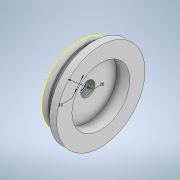
# Autodesk Inventor part: Крышка_пром_новая
Saved by Autodesk Inventor 2021 (Build 250183000, 183)
## iProperties
Created: 2023-04-26
Part Number: Крышка_пром_новая
Material: Типовые
Document SubType Name: Modeling
Designer: gdevc
Density: 1 g/cm^3
Appearance: По умолчанию
Mass: 23.6279 g
Surface Area: 96.7653 cm^2
Volume: 23.6279 cm^3
Author: gdevc
Autodesk Inventor part; units mm, degrees
ref_plane "YZ Plane" through (0, 0, 0) normal (1, 0, 0) x (0, 1, 0)
ref_plane "XZ Plane" through (0, 0, 0) normal (0, 1, 0) x (-1, 0, 0)
ref_plane "XY Plane" through (0, 0, 0) normal (0, 0, 1) x (1, 0, 0)
sketch "Эскиз1" plane through (0, 0, 0) normal (0, 0, 1) x (1, 0, 0)
  line L0 (0, 0) -> (0, 26)
  line L1 (10, 26.1456) -> (10, 30.5)
  line L2 (10, 30.5) -> (15, 30.5)
  line L3 (15, 30.5) -> (15, 20)
  line L4 (15, 20) -> (6, 20)
  line L5 (6, 20) -> (6, 0)
  line L6 (6, 0) -> (0, 0)
  line L7 (0, 26) -> (4.5, 26)
  line L8 (4.5, 26) -> (5, 25.5)
  line L9 (5, 25.5) -> (10, 25.5)
  line L10 (10, 25.5) -> (10, 26.1456)
  dimension "d1" = 52
  dimension "d2" = 0.5
  dimension "d3" = 45
  dimension "d4" = 5
  dimension "d5" = 15
  dimension "d6" = 6
  dimension "d7" = 40
  dimension "d8" = 4.5
  dimension "d23" = 10
  constraints: 22 end point, 6 perpendicular, 1 horizontal, 1 parallel, 1 vertical
  measures "d1" diameter of L7 L6
  measures "d2" distance between parallel lines of L7 L9
  measures "d3" angle of L7 L8
  measures "d4" distance of L8.end L9.end
  measures "d5" distance between parallel lines of L3 L0
  measures "d6" distance between parallel lines of L0 L5
  measures "d7" diameter of L4 L6
  measures "d8" distance between parallel lines of L7 L2
  measures "d23" distance between parallel lines of L0 L1
revolve "Вращение1" add sketch "Эскиз1" angle 360 about axis through (6, 0, 0) along (-1, 0, 0)
sketch "Эскиз2" plane through (0, 0, 0) normal (-1, 0, 0) x (0, 0, 1)
  circle A0 centre (0, 0) radius 26 projected
  circle A1 centre (0, 0) radius 10
  circle A2 centre (0, 0) radius 5
  point P0 (0, 0)
  dimension "d10" = 20
  dimension "d11" = 10
  constraints: 2 centre point, 2 coincident
  measures "d10" diameter of A1
  measures "d11" diameter of A2
extrude "Выдавливание1" cut sketch "Эскиз2" against normal through all contours A2
fillet "Сопряжение2" radius 0.5 1 edges at (5, -25.5, 0)
thread "Резьба2" size "M10x1.5" class "6H" standard "ANSI Metric M Profile" length 10
chamfer "Фаска2" distance 1 angle 45 1 edges at (0, 0, -5)
